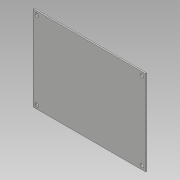
# Autodesk Inventor part: 基板
Saved by Autodesk Inventor 2017 (Build 210142000, 142)
## iProperties
Part Number: 基板
Material: 一般
Document SubType Name: Modeling
Designer: HISAAKI
Density: 1 g/cm^3
Appearance: 既定
Author: HISAAKI
Autodesk Inventor part; units mm, degrees
ref_plane "YZ Plane" through (0, 0, 0) normal (1, 0, 0) x (0, 1, 0)
ref_plane "XZ Plane" through (0, 0, 0) normal (0, 1, 0) x (-1, 0, 0)
ref_plane "XY Plane" through (0, 0, 0) normal (0, 0, 1) x (1, 0, 0)
sketch "スケッチ1" plane through (0, 0, 0) normal (0, 1, 0) x (-1, 0, 0)
  line L0 (0, 0) -> (95, 0)
  line L1 (95, 0) -> (95, -72)
  line L2 (95, -72) -> (0, -72)
  line L3 (0, -72) -> (0, 0)
  dimension "d0" = 95
  dimension "d1" = 72
  constraints: 8 end point, 2 parallel, 1 horizontal, 1 perpendicular
  measures "d0" distance of L1.end L2.end
  measures "d1" distance of L0.end L1.end
extrude "押し出し1" add sketch "スケッチ1" along normal blind 1
hole "穴1" at (-92, 1, -3) direction (0, -1, 0) diameter 3 end through all
hole "穴2" at (-92, 1, -69) direction (0, -1, 0) diameter 3 end through all
hole "穴3" at (-3, 1, -3) direction (0, -1, 0) diameter 3 end through all
hole "穴4" at (-3, 1, -69) direction (0, -1, 0) diameter 3 end through all
